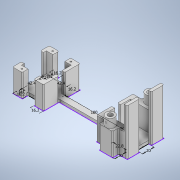
# Autodesk Inventor part: Hold of motors
Saved by Autodesk Inventor 2022 (Build 260153000, 153)
## iProperties
Created: 2021-12-30
Part Number: Hold of motors
Material: Generic
Document SubType Name: Modeling
Designer: simon
Density: 1 g/cm^3
Appearance: Default
Author: simon
Autodesk Inventor part; units mm, degrees
ref_plane "YZ Plane" through (0, 0, 0) normal (1, 0, 0) x (0, 1, 0)
ref_plane "XZ Plane" through (0, 0, 0) normal (0, 1, 0) x (-1, 0, 0)
ref_plane "XY Plane" through (0, 0, 0) normal (0, 0, 1) x (1, 0, 0)
sketch "Sketch1" plane through (0, 0, 0) normal (0, 1, 0) x (-1, 0, 0)
  line L0 (-21.2, 21.2) -> (21.2, 21.2)
  line L1 (21.2, 21.2) -> (21.2, -21.2)
  line L2 (21.2, -21.2) -> (-21.2, -21.2)
  line L3 (-21.2, -21.2) -> (-21.2, 21.2)
  line L4 (-21.2, 21.2) -> (21.2, -21.2) construction
  line L5 (21.2, 21.2) -> (-21.2, -21.2) construction
  line L6 (26.2, 26.2) -> (26.2, 31.2)
  line L7 (26.2, -26.2) -> (26.2, -31.2)
  line L8 (-26.2, 26.2) -> (-26.2, 31.2)
  line L9 (-26.2, -26.2) -> (-26.2, -31.2)
  line L10 (26.2, 31.2) -> (10, 31.2)
  line L11 (10, 31.2) -> (10, 21.2)
  line L12 (-26.2, 31.2) -> (-10, 31.2)
  line L13 (-10, 31.2) -> (-10, 21.2)
  line L14 (-26.2, -31.2) -> (-10, -31.2)
  line L15 (-10, -31.2) -> (-10, -21.2)
  line L16 (26.2, -31.2) -> (10, -31.2)
  line L17 (10, -31.2) -> (10, -21.2)
  line L18 (26.2, 31.2) -> (26.2, 16.2)
  line L19 (26.2, 16.2) -> (21.2, 16.2)
  line L20 (26.2, -31.2) -> (26.2, -16.2)
  line L21 (26.2, -16.2) -> (21.2, -16.2)
  line L22 (26.2, 31.2) -> (10, 31.2)
  line L23 (-10, 31.2) -> (-26.2, 31.2)
  line L24 (26.2, -26.2) -> (26.2, -16.2)
  line L25 (26.2, 16.2) -> (26.2, 26.2)
  line L26 (-26.2, -31.2) -> (-10, -31.2)
  line L27 (10, -31.2) -> (26.2, -31.2)
  line L28 (-21.2, 5) -> (-121.2, 5)
  line L29 (-121.2, 5) -> (-121.2, -5)
  line L30 (-121.2, -5) -> (-21.2, -5)
  line L31 (-21.2, -5) -> (-21.2, 5)
  line L32 (-71.2, -5) -> (-71.2, 5)
  line L33 (-121.2, 21.2) -> (-163.6, 21.2)
  line L34 (-163.6, 21.2) -> (-163.6, -21.2)
  line L35 (-163.6, -21.2) -> (-121.2, -21.2)
  line L36 (-121.2, -21.2) -> (-121.2, 21.2)
  line L37 (-116.2, 26.2) -> (-116.2, 31.2)
  line L38 (-116.2, -26.2) -> (-116.2, -31.2)
  line L39 (-116.2, 31.2) -> (-131, 31.2)
  line L40 (-116.2, 26.2) -> (-116.2, 5)
  line L41 (-116.2, -5) -> (-116.2, -26.2)
  line L42 (-26.2, 26.2) -> (-26.2, 5)
  line L43 (-26.2, -5) -> (-26.2, -26.2)
  line L44 (-116.2, 26.2) -> (-116.2, -26.2)
  line L45 (-163.6, 10) -> (-168.6, 10)
  line L46 (-168.6, -10) -> (-163.6, -10)
  line L47 (-131, 41.2) -> (-153.8, 41.2)
  line L48 (-153.8, 41.2) -> (-153.8, 21.2)
  line L49 (-153.8, 21.2) -> (-131, 21.2)
  line L50 (-131, 21.2) -> (-131, 41.2)
  line L51 (-131, 41.2) -> (-153.8, 21.2) construction
  line L52 (-153.8, 41.2) -> (-131, 21.2) construction
  line L53 (-168.6, 31.2) -> (-153.8, 31.2)
  line L54 (-131, 31.2) -> (-116.2, 31.2)
  line L55 (-121.2, 0) -> (-158.6, 0)
  line L56 (-121.2, -21.2) -> (-163.6, -21.2)
  line L57 (-116.2, -31.2) -> (-131, -31.2)
  line L58 (-153.8, -41.2) -> (-153.8, -21.2)
  line L59 (-131, -21.2) -> (-131, -41.2)
  line L60 (-168.6, -31.2) -> (-153.8, -31.2)
  line L61 (-168.6, -31.2) -> (-168.6, -25.8352)
  line L62 (-168.6, 31.2) -> (-168.6, 26.2)
  line L63 (-131, -41.2) -> (-153.8, -41.2)
  line L64 (-168.6, -26.2) -> (-168.6, -10)
  line L65 (-168.6, 10) -> (-168.6, 26.2)
  line L66 (-163.6, 21.2) -> (-163.6, 31.2)
  line L67 (-163.6, -21.2) -> (-163.6, -31.2)
  point P0 (0, 0)
  point P1 (-163.6, 0)
  point P2 (-121.2, -5)
  point P3 (-21.2, -5)
  point P4 (-121.2, 5)
  dimension "d0" = 42.4
  dimension "d1" = 42.4
  dimension "d4" = 16.2
  dimension "d5" = 16.2
  dimension "d6" = 16.2
  dimension "d7" = 16.2
  dimension "d8" = 15
  dimension "d9" = 15
  dimension "d12" = 100
  dimension "d16" = 20
  dimension "d17" = 22.8
  dimension "d18" = 20
  constraints: 136 end point, 21 point on line, 15 parallel, 15 symmetric about line, 11 perpendicular, 10 midpoint, 5 horizontal, 1 vertical
  measures "d0" distance of L1.end L2.end
  measures "d1" distance of L0.end L1.end
  measures "d4" distance of L6.end L10.end
  measures "d5" distance of L8.end L12.end
  measures "d6" distance of L9.end L14.end
  measures "d7" distance of L7.end L16.end
  measures "d8" distance of L6.end L18.end
  measures "d9" distance of L7.end L20.end
  measures "d12" distance of L30.end L29.end
  measures "d16" distance of L46.start L45.end
  measures "d17" distance of L49.end L48.end
  measures "d18" distance of L48.end L47.end
extrude "Extrusion1" add sketch "Sketch1" along normal blind 5 contours L0 L1 L2 L3 | L3 L30 L32 L28 | L32 L30 L44 L28 | L44 L30 L29 L28 | L29 L36 L35 L34 L33
extrude "Extrusion2" add sketch "Sketch1" along normal blind 38.8 contours L3 L28 L42 L8 L12 L13 L0 | L11 L10 L6 L18 L19 L1 L0 | L3 L2 L15 L14 L9 L43 L30 | L21 L20 L7 L16 L17 L2 L1
extrude "Extrusion3" add sketch "Sketch1" along normal blind 38.8 contours L28 L36 L33 L50 L39 L37 L40 | L41 L38 L57 L59 L35 L36 L30 | L33 L48 L47 L50 | L59 L63 L58 L35 | L33 L66 L53 L48 | L58 L60 L67 L35
extrude "Extrusion4" add sketch "Sketch1" along normal blind 78.8 contours L34 L45 L65 L62 L53 L66 | L67 L60 L61 L64 L46 L34
sketch "Sketch2" plane through (0, 38.8, 0) normal (0, 1, 0) x (1, 0, 0)
  line L0 (10, -21.2) -> (10, -31.2) projected
  line L1 (10, -26.2) -> (14.3, -26.2)
  line L2 (14.3, -26.2) -> (15.55, -26.2)
  circle A0 centre (15.55, -26.2) radius 1.25
  line L3 (-10, -21.2) -> (10, -21.2) projected
  line L4 (0, -21.2) -> (0, 21.2)
  line L5 (10, 21.2) -> (-10, 21.2) projected
  circle A1 centre (-15.55, -26.2) radius 1.25
  line L6 (-21.2, 16.2) -> (-21.2, -16.2) projected
  line L7 (-21.2, 0) -> (21.2, 0)
  circle A2 centre (15.55, 26.2) radius 1.25
  circle A3 centre (-15.55, 26.2) radius 1.25
  line L8 (116.2, 5) -> (26.2, 5) projected
  line L9 (71.2, 5) -> (71.2, -5)
  line L10 (26.2, -5) -> (116.2, -5) projected
  circle A4 centre (126.85, -26.2) radius 1.25
  circle A5 centre (157.95, -26.2) radius 1.25
  circle A6 centre (157.95, 26.2) radius 1.25
  circle A7 centre (126.85, 26.2) radius 1.25
  point P0 (0, 0)
  dimension "d27" = 4.3
  dimension "d28" = 1.25
  dimension "d29" = 2.5
  constraints: 10 end point, 8 centre point, 8 symmetric about line, 6 midpoint, 3 horizontal, 2 coincident, 7 other
  measures "d27" distance of L1.start L1.end
  measures "d28" distance of L1.end L2.end
  measures "d29" diameter of A0
extrude "Extrusion5" cut sketch "Sketch2" against normal blind 5
sketch "Sketch3" plane through (0, 38.8, 0) normal (0, 1, 0) x (1, 0, 0)
  line L0 (131, -41.2) -> (153.8, -41.2) projected
  line L1 (142.4, -41.2) -> (142.4, -33.7)
  circle A0 centre (142.4, -33.7) radius 7.5
  circle A1 centre (142.4, -33.7) radius 4.05
  line L2 (163.6, -10) -> (163.6, 10) projected
  line L3 (163.6, 0) -> (121.2456, 0)
  circle A2 centre (142.4, 33.7) radius 7.5
  circle A3 centre (142.4, 33.7) radius 4.05
  point P0 (0, 0)
  dimension "d32" = 7.5
  dimension "d33" = 8.1
  constraints: 4 end point, 3 centre point, 3 coincident, 2 midpoint, 2 symmetric about line, 1 horizontal, 1 vertical, 1 vertical alignment, 4 other
  measures "d32" distance of L1.start L1.end
  measures "d33" diameter of A1
extrude "Extrusion6" add sketch "Sketch3" along normal blind 15
sketch "Sketch4" plane through (131, 0, 41.2) normal (0, 0, 1) x (1, 0, 0)
  line L0 (18.9, 53.8) -> (3.9, 53.8) projected
  line L1 (3.9, 38.8) -> (18.9, 38.8) projected
  line L2 (18.9, 53.8) -> (3.9, 53.8) projected
  line L3 (22.8, 38.8) -> (11.4, 38.8) projected
  line L4 (11.4, 53.8) -> (11.4, 38.8)
  circle A0 centre (11.4, 46.3) radius 1.25
  point P0 (-131, 0)
  dimension "d36" = 2.5
  constraints: 2 end point, 2 midpoint, 1 centre point, 1 vertical
  measures "d36" diameter of A0
extrude "Extrusion7" cut sketch "Sketch4" against normal blind 5
sketch "Sketch5" plane through (153.8, 0, -41.2) normal (0, 0, -1) x (-1, 0, 0)
  line L0 (18.9, 53.8) -> (3.9, 53.8) projected
  line L1 (3.9, 38.8) -> (18.9, 38.8) projected
  line L2 (11.4, 38.8) -> (22.8, 38.8) projected
  line L3 (11.4, 38.8) -> (11.4, 53.8)
  line L4 (7.35, 53.8) -> (15.45, 53.8) projected
  circle A0 centre (11.4, 46.3) radius 1.25
  point P0 (153.8, 0)
  dimension "d39" = 2.5
  constraints: 2 end point, 2 midpoint, 1 centre point
  measures "d39" diameter of A0
extrude "Extrusion8" cut sketch "Sketch5" against normal blind 5
fillet "Fillet1" radius 2 7 edges at (-26.2, 19.4, -31.2) (-26.2, 19.4, -16.2) (-10, 19.4, -31.2) (10, 19.4, -31.2) (26.2, 19.4, -31.2) (26.2, 21.9, -5) (26.2, 2.5, -5)
fillet "Fillet2" radius 2 11 edges at (-26.2, 19.4, 16.2) (-21.2, 2.5, 16.2) (-21.2, 2.5, -16.2) (-26.2, 19.4, 31.2) (-10, 19.4, 31.2) (-10, 2.5, 21.2) (10, 19.4, 31.2) (26.2, 19.4, 31.2) (26.2, 2.5, 5) (26.2, 21.9, 5) (10, 2.5, 21.2)
fillet "Fillet3" radius 2 18 edges at (153.8, 19.4, 31.2) (153.8, 19.4, 41.2) (131, 19.4, 41.2) (131, 19.4, 31.2) (116.2, 19.4, 31.2) (116.2, 2.5, 5) (116.2, 21.9, -5) (116.2, 21.9, 5) (116.2, 2.5, -5) (116.2, 19.4, -31.2) (131, 19.4, -31.2) (131, 19.4, -41.2) (153.8, 19.4, -31.2) (153.8, 19.4, -41.2) (168.6, 39.4, -31.2) (168.6, 39.4, 10) (168.6, 39.4, -10) (168.6, 39.4, 31.2)
body "Solid1"
